3D Printing Tuning (Autodesk Fusion 360 design; units mm, degrees)
Autodesk Fusion 360 part; units mm, degrees
note: some values were not read from the file. Chosen so that the rebuilt part matches the saved one: the sign of a taper.
sketch "Bridging Test" plane through (0, 0, 0) normal (1, 0, 0) x (0, 1, 0) in component "Bridging Test"
  line L0 (-10, 10) -> (-10, 0)
  line L1 (-10, 0) -> (-15, 0)
  line L2 (-15, 0) -> (-11, 10.4)
  line L3 (-10, 10) -> (10, 10)
  line L4 (-11, 10.4) -> (11, 10.4)
  line L5 (0, 2.5) -> (0, 20) construction
  line L6 (15, 0) -> (11, 10.4)
  line L7 (10, 0) -> (15, 0)
  line L8 (10, 10) -> (10, 0)
  dimension "d1" = 5
  dimension "d2" = 10
  dimension "d3" = 0.4
  dimension "d4" = 1
  dimension "d5" = 20
  constraint vertical L0
  constraint perpendicular L0 L1
  constraint perpendicular L0 L3
  constraint horizontal L4
  constraint coincident origin L1
  constraint symmetric L0.start L5 L3.end
  constraint symmetric L0.end L5 L7.start
  constraint symmetric L1.end L5 L6.start
  constraint symmetric L2.end L5 L4.end
  constraint coincident L3.end L8.start
  constraint coincident L4.end L6.end
  measures "d1" distance of L0.end L1.end
  measures "d2" distance of L0.start L0.end
  measures "d3" vertical distance of L0.start L2.end
  measures "d4" horizontal distance of L0.start L2.end
  measures "d5" distance of L0.start L3.end
extrude "Extrude1" add sketch "Bridging Test" along normal blind 7 makes body 1 in component "Bridging Test"
sketch "Sketch1" plane through (0, 0, 0) normal (0, 0, 1) x (1, 0, 0) in component "Stringing test"
  line L0 (-40, 0.8) -> (-44, 0.8)
  line L1 (-40, 0.8) -> (-40, 0)
  line L2 (-40, 0) -> (-43.2, 0)
  line L3 (-43.2, 0) -> (-43.2, -3.2)
  line L4 (-43.2, -3.2) -> (-44, -3.2)
  line L5 (-44, -3.2) -> (-44, 0.8)
  line L6 (-40, 0.8) -> (0, 0.8)
  line L7 (0, 0.8) -> (0, 0)
  line L8 (0, 0) -> (-40, 0)
  dimension "d12" = 4
  dimension "d13" = 4
  dimension "d16" = 0.8
  dimension "d17" = 40
  constraint horizontal L7.end L1.end
  constraint perpendicular L0 L1
  constraint perpendicular L1 L2
  constraint perpendicular L2 L3
  constraint perpendicular L4 L5
  constraint equal L1 L4
  constraint horizontal L0
  constraint vertical L5
  constraint perpendicular L1 L6
  constraint coincident L7.end L8.start
  constraint equal L6 L8
  measures "d12" distance of L0.end L4.end
  measures "d13" distance of L0.start L0.end
  measures "d16" distance of L1.end L0.start
  measures "d17" distance of L7.end L1.end
extrude "Extrude1'" add sketch "Sketch1" along normal blind 20 separate body contours L0 L1 L2 L3 L4 L5 makes body 2 in component "Stringing test"
draft "Draft1" angle 8 neutral plane through (0, 0, 0) pull (0, 0, 1) 2 faces at (-43.4667, -3.2, 6.6667) (-40, 0.5333, 6.6667) on bodies 2 in component "Stringing test"
extrude "Extrude2" add sketch "Sketch1" along normal blind 0.2 separate body contours L1 L6 L7 L8 makes body 3 in component "Stringing test"
mirror "Mirror2" about plane through (0, 0, 0) normal (1, 0, 0) of bodies 2 3 makes body 4 at (42.2703, 0.8, 6.6667) makes body 5 at (13.3333, 0.5333, 0) in component "Stringing test"
combine "Combine1" operation add target body 2 tool bodies 3 5 4 in component "Stringing test"
sketch "Sketch1 (2)" plane through (0, 0, 0) normal (0, 1, 0) x (1, 0, 0) in component "Temperature tower"
  line L0 (-10, -9) -> (49, -9)
  line L1 (49, -9) -> (40, 0)
  line L2 (40, 0) -> (35, 0)
  line L3 (35, 0) -> (35, -8.4)
  line L4 (35, -8.4) -> (5, -8.4)
  line L5 (5, -8.4) -> (5, 0)
  line L6 (5, 0) -> (0, 0)
  line L7 (0, 0) -> (-4.9786, 0) construction
  line L8 (0, 0) -> (0, -4.4978) construction
  line L9 (40, 0) -> (40, -4.4978) construction
  line L10 (0, 0) -> (0, -3.2265)
  line L11 (0, -3.2265) -> (-10, -9)
  dimension "d24" = 5
  dimension "d26" = 0.6
  dimension "d28" = 45
  dimension "d29" = 60
  dimension "d30" = 10
  dimension "d31" = 5
  dimension "d32" = 9
  dimension "d33" = 30
  constraint horizontal L0
  constraint parallel L0 L2
  constraint perpendicular L2 L3
  constraint perpendicular L3 L4
  constraint perpendicular L4 L5
  constraint coincident L6.end L7.start
  constraint perpendicular L5 L6
  constraint parallel L6 L7
  constraint perpendicular L7 L8
  constraint perpendicular L2 L9
  constraint coincident L8 L10.end
  constraint collinear L2 L6
  measures "d24" distance of L5.end L6.end
  measures "d26" distance of L0 L4
  measures "d28" angle of L1 L9
  measures "d29" angle of L8 L11
  measures "d30" distance of L10 L0.start
  measures "d31" distance of L1.end L2.end
  measures "d32" distance of L0 L6.end
  measures "d33" distance of L3.end L4.end
extrude "Extrude1''" add sketch "Sketch1 (2)" along normal blind 8 separate body makes body 6 in component "Temperature tower"
move_face "MoveFace1" to x (0.965926, 0.258819, 0) y (-0.258819, 0.965926, 0) z (0, 0, 1) at (1.2056, -1.1578, 0) 1 faces at (5, 2.6667, 5.6) on bodies 6 in component "Temperature tower"
move_face "MoveFace2" to x (0.965926, -0.258819, 0) y (0.258819, 0.965926, 0) z (0, 0, 1) at (-0.0131, 7.9009, 0) 1 faces at (35, 2.6667, 2.8) on bodies 6 in component "Temperature tower"
pattern_linear "R-Pattern1" count 5 spacing 9 along (0, 0, 1) of bodies 6 makes body 7 at (9.6667, 5.3333, 18) makes body 8 at (9.6667, 5.3333, 27) makes body 9 at (9.6667, 5.3333, 36) makes body 10 at (9.6667, 5.3333, 45) in component "Temperature tower"
combine "Combine1'" operation add target body 9 tool bodies 8 6 7 10 in component "Temperature tower"
component "Bridging Test" placed x (1, 0, 0) y (0, 1, 0) z (0, 0, 1) at (0, 0, 0)
component "Stringing test" placed x (1, 0, 0) y (0, 1, 0) z (0, 0, 1) at (0, 0, 0)
component "Temperature tower" placed x (1, 0, 0) y (0, 1, 0) z (0, 0, 1) at (0, 0, 0)
named bodies: "Stringing Test", "Temp Tower"
